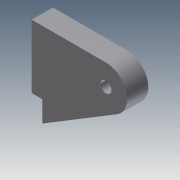
# Autodesk Inventor part: linacconnectspecial top
Saved by Autodesk Inventor 2011 (Build 150239000, 239)
## iProperties
Created: 2011-01-02
Part Number: linacconnectspecial top
Document SubType Name: Modeling
Designer: Matthew
Density: 1 g/cm^3
Author: Matthew
Autodesk Inventor part; units mm, degrees
ref_plane "YZ Plane" through (0, 0, 0) normal (1, 0, 0) x (0, 1, 0)
ref_plane "XZ Plane" through (0, 0, 0) normal (0, 1, 0) x (-1, 0, 0)
ref_plane "XY Plane" through (0, 0, 0) normal (0, 0, 1) x (1, 0, 0)
sketch "Sketch1" plane through (0, 0, 0) normal (0, 0, 1) x (1, 0, 0)
  line L0 (-18.1672, 18.8103) -> (-11.8172, 18.8103)
  line L1 (-11.8172, 18.8103) -> (-11.8172, -19.2897)
  line L2 (-11.8172, -19.2897) -> (-18.1672, -19.2897)
  line L3 (-18.1672, -19.2897) -> (-18.1672, 18.8103)
  line L4 (-11.8172, 18.8103) -> (32.6328, 18.8103)
  line L5 (-11.8172, -19.2897) -> (-11.8172, -25.6397)
  line L6 (-11.8172, 18.8103) -> (-11.8172, 6.1103)
  line L7 (-11.8172, 6.1103) -> (26.3844, 6.1103)
  circle A0 centre (26.3844, 6.1103) radius 3.3
  circle A1 centre (26.3844, 6.1103) radius 12.7
  line L8 (-18.1672, 18.8103) -> (26.3844, 18.8103)
  line L9 (-11.8172, -25.6397) -> (-11.8172, -31.9897)
  line L10 (-11.8172, -31.9897) -> (32.984, -4.7403)
  point P0 (0, 0)
  dimension "d0" = 6.35
  dimension "d1" = 38.1
  dimension "d2" = 44.45
  dimension "d3" = 6.35
  dimension "d4" = 12.7
  dimension "d5" = 38.2016
  dimension "d6" = 6.6
  dimension "d7" = 6.35
  constraints: 22 end point, 5 perpendicular, 2 centre point, 2 coincident, 2 parallel, 2 point on circle, 2 point on line, 2 tangent, 1 horizontal
  measures "d0" distance of L1.end L2.end
  measures "d1" distance of L0.end L1.end
  measures "d2" distance of L0.end L4.end
  measures "d3" distance of L1.end L5.end
  measures "d4" distance of L0.end L6.end
  measures "d5" distance of L6.end L7.end
  measures "d6" diameter of A0
  measures "d7" distance of L5.end L9.end
extrude "Extrusion1" add sketch "Sketch1" along normal blind 12.7
body "Solid1"
